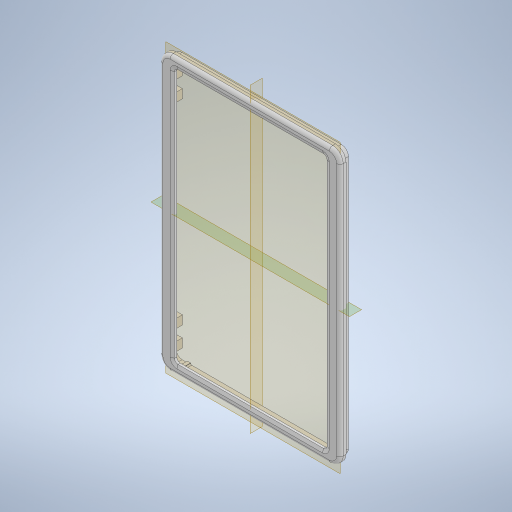
# Autodesk Inventor part: front-bezel
Saved by Autodesk Inventor 2024 (Build 280153000, 153)
## iProperties
Created: 2024-11-23
Part Number: front-bezel
Material: Generic
Document SubType Name: Modeling
Designer: Stefano
Density: 1 g/cm^3
Appearance: Default
Author: Stefano
Autodesk Inventor part; units mm, degrees
ref_plane "YZ Plane" through (0, 0, 0) normal (1, 0, 0) x (0, 1, 0)
ref_plane "XZ Plane" through (0, 0, 0) normal (0, 1, 0) x (-1, 0, 0)
ref_plane "Work Plane1" through (0, 0, 0) normal (0, 0, 1) x (1, 0, 0)
sketch "Sketch1" plane through (0, 0, 0) normal (0, 0, 1) x (1, 0, 0)
  line L0 (71.25, 117.5) -> (71.25, -117.5) construction
  line L1 (-71.25, 117.5) -> (71.25, 117.5) construction
  line L2 (-71.25, -117.5) -> (-71.25, 117.5) construction
  line L3 (71.25, -117.5) -> (-71.25, -117.5) construction
  line L4 (68.71, -114.96) -> (68.71, 114.96)
  line L5 (68.71, 114.96) -> (-68.71, 114.96)
  line L6 (-68.71, 114.96) -> (-68.71, -114.96)
  line L7 (-68.71, -114.96) -> (68.71, -114.96)
  line L8 (81.25, 123.5) -> (-81.25, 123.5)
  line L9 (-81.25, 123.5) -> (-81.25, -123.5)
  line L10 (-81.25, -123.5) -> (81.25, -123.5)
  line L11 (81.25, -123.5) -> (81.25, 123.5)
  point P0 (0, 0)
  dimension "d0" = 2.54
  dimension "d1" = 10
  dimension "d3" = 6
  dimension "d4" = 6
  dimension "d12" = 10
  constraints: 16 end point, 2 parallel, 1 horizontal, 1 perpendicular, 3 other
  measures "d0" distance between parallel lines of L0 L4
  measures "d1" distance between parallel lines of L11 L0
  measures "d3" distance between parallel lines of L8 L1
  measures "d4" distance between parallel lines of L3 L10
  measures "d12" distance between parallel lines of L9 L2
extrude "Extrusion1" add sketch "Sketch1" along normal blind 3
fillet "Fillet1" radius 9.525 4 edges at (81.25, 123.5, 1.5) (-81.25, 123.5, 1.5) (-81.25, -123.5, 1.5) (81.25, -123.5, 1.5)
sketch "Sketch2" plane through (0, 0, 0) normal (0, 0, -1) x (-1, 0, 0)
  arc A0 (-81.25, -113.975) -> (-71.725, -123.5) centre (-71.725, -113.975) ccw construction
  line L0 (71.725, -123.5) -> (-71.725, -123.5) construction
  arc A1 (71.725, -123.5) -> (81.25, -113.975) centre (71.725, -113.975) ccw construction
  line L1 (81.25, 113.975) -> (81.25, -113.975) construction
  arc A2 (81.25, 113.975) -> (71.725, 123.5) centre (71.725, 113.975) ccw construction
  line L2 (-71.725, 123.5) -> (71.725, 123.5) construction
  arc A3 (-71.725, 123.5) -> (-81.25, 113.975) centre (-71.725, 113.975) ccw construction
  line L3 (-81.25, -113.975) -> (-81.25, 113.975) construction
  line L4 (-68.71, -114.96) -> (68.71, -114.96) construction
  line L5 (-68.71, 114.96) -> (-68.71, -114.96) construction
  line L6 (68.71, 114.96) -> (-68.71, 114.96) construction
  line L7 (68.71, -114.96) -> (68.71, 114.96) construction
  arc A4 (71.725, -120.3) -> (78.05, -113.975) centre (71.725, -113.975) ccw
  line L8 (71.725, -120.3) -> (-71.725, -120.3)
  arc A5 (-78.05, -113.975) -> (-71.725, -120.3) centre (-71.725, -113.975) ccw
  line L9 (-78.05, -113.975) -> (-78.05, 113.975)
  arc A6 (-71.725, 120.3) -> (-78.05, 113.975) centre (-71.725, 113.975) ccw
  line L10 (-71.725, 120.3) -> (71.725, 120.3)
  arc A7 (78.05, 113.975) -> (71.725, 120.3) centre (71.725, 113.975) ccw
  line L11 (78.05, 113.975) -> (78.05, -113.975)
  arc A8 (71.725, -119.3) -> (77.05, -113.975) centre (71.725, -113.975) ccw
  line L12 (71.725, -119.3) -> (-71.725, -119.3)
  arc A9 (-77.05, -113.975) -> (-71.725, -119.3) centre (-71.725, -113.975) ccw
  line L13 (-77.05, -113.975) -> (-77.05, 113.975)
  arc A10 (-71.725, 119.3) -> (-77.05, 113.975) centre (-71.725, 113.975) ccw
  line L14 (-71.725, 119.3) -> (71.725, 119.3)
  arc A11 (77.05, 113.975) -> (71.725, 119.3) centre (71.725, 113.975) ccw
  line L15 (77.05, 113.975) -> (77.05, -113.975)
  point P0 (0, 0)
  dimension "d8" = 3.2
  dimension "d9" = 1
  constraints: 16 end point, 16 point on circle, 8 centre point, 14 other
  measures "d8" distance between parallel lines of L1 L11
  measures "d9" radial gap between concentric circles of A4 A8
ref_plane "Work Plane2" through (-71.25, -117.5, -7.874) normal (0, 0, -1) x (0, 1, 0)
extrude "Extrusion2" add sketch "Sketch2" along normal up to surface (7.874 mm away)
sketch "Sketch3" plane through (0, 0, 0) normal (0, 0, -1) x (-1, 0, 0)
  circle A0 centre (-73.6832, -106.1863) radius 2 construction
  line L0 (-71.25, 117.5) -> (-71.25, -117.5) construction
  line L1 (-71.25, -117.5) -> (71.25, -117.5) construction
  line L2 (-77.05, 113.975) -> (-77.05, -113.975) projected
  line L3 (-71.25, -110.1863) -> (-77.05, -110.1863)
  line L4 (-77.05, -110.1863) -> (-77.05, -102.1863)
  line L5 (-77.05, -102.1863) -> (-71.25, -102.1863)
  line L6 (-71.25, -102.1863) -> (-71.25, -110.1863)
  line L7 (-71.725, -119.3) -> (71.725, -119.3) projected
  line L8 (-67.05, -117.5) -> (-64.05, -117.5)
  line L9 (-64.05, -117.5) -> (-64.05, -119.3)
  line L10 (-64.05, -119.3) -> (-67.05, -119.3)
  line L11 (-67.05, -119.3) -> (-67.05, -117.5)
  line L12 (-71.504, -102.1863) -> (-71.504, -110.1863)
  line L13 (-77.05, -92.1863) -> (-71.504, -92.1863)
  line L14 (-71.504, -92.1863) -> (-71.504, -84.1863)
  line L15 (-71.504, -84.1863) -> (-77.05, -84.1863)
  line L16 (-77.05, -84.1863) -> (-77.05, -92.1863)
  line L17 (-77.05, -84.1863) -> (-71.504, -92.1863) construction
  circle A1 centre (-74.277, -88.1863) radius 1.5
  line L18 (-67.05, -118.008) -> (-64.05, -118.008)
  point P0 (0, 0)
  dimension "d13" = 4
  dimension "d14" = 4
  dimension "d15" = 10
  dimension "d16" = 3
  dimension "d28" = 0.254
  dimension "d34" = 10
  dimension "d35" = 8
  dimension "d36" = 3
  dimension "d45" = 0.508
  constraints: 30 end point, 9 point on line, 6 parallel, 5 perpendicular, 3 horizontal, 1 centre point, 1 collinear, 1 midpoint
  measures "d13" distance from line of L5 A0.centre
  measures "d14" distance from line of A0.centre L3
  measures "d15" distance between parallel lines of L11 L2
  measures "d16" distance between parallel lines of L11 L9
  measures "d28" distance between parallel lines of L12 L6
  measures "d34" distance between parallel lines of L13 L5
  measures "d35" distance between parallel lines of L13 L15
  measures "d36" diameter of A1
  measures "d45" distance between parallel lines of L8 L18
extrude "Extrusion3" add sketch "Sketch3" along normal up to surface (7.874 mm away) contours L15 L14 L13 L2 | L5 L12 L3 L2 | L11 L18 L9 L7
chamfer "Chamfer2" distance 5.08 distance2 0.508 1 edges at (65.55, -118.008, -7.874) measured on face at (65.55, -118.008, -7.374)
sketch "Sketch5" plane through (71.725, -120.3, -7.874) normal (0, 0, -1) x (-1, 0, 0)
  point P0 (71.725, 120.3)
  point P1 (-1.9582, 14.1137)
hole "Hole1" at (73.6832, -106.1863, -7.874) direction (0, 0, 1) diameter 3 depth 6.35
ref_plane "Work Plane3" through (-71.725, 0, 0) normal (0, -1, 0) x (1, 0, 0)
ref_plane "Work Plane4" through (0, -113.975, 0) normal (1, 0, 0) x (0, 0, -1)
mirror "Mirror1" about plane through (-71.725, 0, 0) normal (0, -1, 0) of "Extrusion3", "Hole1", "Chamfer2"
mirror "Mirror2" about plane through (0, -113.975, 0) normal (1, 0, 0) of "Extrusion3", "Hole1", "Mirror1"
fillet "Fillet2" radius 3.175 4 edges at (-68.71, -114.96, 1.5) (68.71, -114.96, 1.5) (-68.71, 114.96, 1.5) (68.71, 114.96, 1.5)
chamfer "Chamfer1" distance 3 distance2 1 8 edges at (-68.71, 0, 3) (-67.7801, 114.0301, 3) (0, 114.96, 3) (67.7801, 114.0301, 3) (68.71, 0, 3) (67.7801, -114.0301, 3) (0, -114.96, 3) (-67.7801, -114.0301, 3) measured on face at (68.1336, 114.3836, 3) measured on face at (0, 115.46, 3) measured on face at (-68.1336, 114.3836, 3) measured on face at (-68.1336, -114.3836, 3) measured on face at (68.1336, -114.3836, 3) measured on face at (0, -115.46, 3) measured on face at (69.21, 0, 3) measured on face at (-69.21, 0, 3)
fillet "Fillet3" radius 3 8 edges at (78.4602, -120.7102, 3) (81.25, 0, 3) (78.4602, 120.7102, 3) (0, 123.5, 3) (-78.4602, 120.7102, 3) (-81.25, 0, 3) (-78.4602, -120.7102, 3) (0, -123.5, 3)
sketch "Sketch6" plane through (0, 0, 0) normal (0, 0, -1) x (-1, 0, 0)
  line L0 (-77.05, 84.1863) -> (-77.05, -84.1863) projected
  line L1 (-77.05, -4) -> (-71.504, -4)
  line L2 (-71.504, -4) -> (-71.504, 4)
  line L3 (-71.504, 4) -> (-77.05, 4)
  line L4 (-77.05, 4) -> (-77.05, -4)
  line L5 (113.75, 0) -> (-113.75, 0) construction
  line L6 (-71.504, -84.1863) -> (-71.504, -92.1863) construction
  line L7 (-77.05, -4) -> (-71.504, 4) construction
  circle A0 centre (-74.277, 0) radius 1.5
  point P0 (0, 0)
  dimension "d37" = 8
  dimension "d39" = 3
  constraints: 10 end point, 2 parallel, 1 centre point, 1 collinear, 1 horizontal, 1 midpoint, 1 perpendicular, 1 point on line, 1 other
  measures "d37" distance between parallel lines of L3 L1
  measures "d39" diameter of A0
extrude "Extrusion5" [suppressed]
mirror "Mirror3" [suppressed]
fillet "Fillet4" radius 1 68 edges at (77.05, 110.1863, -3.937) (77.05, 102.1863, -3.937) (77.05, 92.1863, -3.937) (77.05, 84.1863, -3.937) (64.05, 119.3, -3.937) (67.05, 119.3, -3.937) (-64.05, 119.3, -3.937) (-67.05, 119.3, -3.937) (-77.05, 110.1863, -3.937) (-77.05, 102.1863, -3.937) (-77.05, 92.1863, -3.937) (-77.05, 84.1863, -3.937) (-77.05, -102.1863, -3.937) (-77.05, -110.1863, -3.937) (-77.05, -92.1863, -3.937) (-77.05, -84.1863, -3.937) (-64.05, -119.3, -3.937) (-67.05, -119.3, -3.937) (77.05, -84.1863, -3.937) (77.05, -92.1863, -3.937) (77.05, -102.1863, -3.937) (77.05, -110.1863, -3.937) (67.05, -119.3, -3.937) (64.05, -119.3, -3.937) (69.3875, -119.3, 0) (77.05, -112.0806, 0) (75.4903, -117.7403, 0) (77.05, -97.1863, 0) (77.05, 97.1863, 0) (77.05, 112.0806, 0) (77.05, 0, 0) (74.277, -84.1863, 0) (74.277, -92.1863, 0) (74.277, -102.1863, 0) (74.277, -110.1863, 0) (64.05, -118.654, 0) (0, -119.3, 0) (67.05, -118.654, 0) (-64.05, -118.654, 0) (-67.05, -118.654, 0) (-75.4903, -117.7403, 0) (-77.05, -112.0806, 0) (-69.3875, -119.3, 0) (-74.277, -110.1863, 0) (-74.277, -102.1863, 0) (-77.05, -97.1863, 0) (-74.277, -92.1863, 0) (-74.277, -84.1863, 0) (-77.05, 112.0806, 0) (-77.05, 97.1863, 0) (-77.05, 0, 0) (-74.277, 84.1863, 0) (-74.277, 92.1863, 0) (-74.277, 102.1863, 0) (-74.277, 110.1863, 0) (-75.4903, 117.7403, 0) (-69.3875, 119.3, 0) (-67.05, 118.654, 0) (-64.05, 118.654, 0) (0, 119.3, 0) (64.05, 118.654, 0) (67.05, 118.654, 0) (75.4903, 117.7403, 0) (69.3875, 119.3, 0) (74.277, 110.1863, 0) (74.277, 102.1863, 0) (74.277, 92.1863, 0) (74.277, 84.1863, 0)
sketch "Sketch7" plane through (0, 0, 0) normal (0, 0, -1) x (-1, 0, 0)
  arc A0 (-81.25, -113.975) -> (-71.725, -123.5) centre (-71.725, -113.975) ccw projected
  line L0 (71.725, -123.5) -> (-71.725, -123.5) projected
  arc A1 (71.725, -123.5) -> (81.25, -113.975) centre (71.725, -113.975) ccw projected
  line L1 (81.25, 113.975) -> (81.25, -113.975) projected
  arc A2 (81.25, 113.975) -> (71.725, 123.5) centre (71.725, 113.975) ccw projected
  line L2 (-71.725, 123.5) -> (71.725, 123.5) projected
  arc A3 (-71.725, 123.5) -> (-81.25, 113.975) centre (-71.725, 113.975) ccw projected
  line L3 (-81.25, -113.975) -> (-81.25, 113.975) projected
  arc A4 (78.05, 113.975) -> (71.725, 120.3) centre (71.725, 113.975) ccw projected
  line L4 (78.05, 113.975) -> (78.05, -113.975) projected
  arc A5 (71.725, -120.3) -> (78.05, -113.975) centre (71.725, -113.975) ccw projected
  line L5 (71.725, -120.3) -> (-71.725, -120.3) projected
  arc A6 (-78.05, -113.975) -> (-71.725, -120.3) centre (-71.725, -113.975) ccw projected
  line L6 (-78.05, -113.975) -> (-78.05, 113.975) projected
  arc A7 (-71.725, 120.3) -> (-78.05, 113.975) centre (-71.725, 113.975) ccw projected
  line L7 (-71.725, 120.3) -> (71.725, 120.3) projected
  point P0 (0, 0)
extrude "Extrusion6" add sketch "Sketch7" along normal blind 2.5
equation "\"d4\" = d3"
equation "\"d12\" = d1"
equation "\"d14\" = d13"
equation "\"d37\" = d35"
body "Solid1"
